Autodesk Fusion 360 part; units mm, degrees
(part 2 of 2)
sketch "Sketch4 (2)" plane through (0, 0, 0) normal (0, 0, 1) x (1, 0, 0)
  circle A0 centre (-53.2335, 49) radius 1.25
  circle A1 centre (-53.2335, -49) radius 1.25
  line L0 (-62.4835, 47.5) -> (-62.4835, -47.5)
  line L1 (-62.4835, -47.5) -> (-57.8585, -47.5)
  line L2 (-57.8585, -47.5) -> (-57.8585, -50.5)
  line L3 (-57.8585, -50.5) -> (-48.6085, -50.5)
  line L4 (-48.6085, -50.5) -> (-48.6085, -47.5)
  line L5 (-48.6085, -47.5) -> (-43.9835, -47.5)
  line L6 (-43.9835, -47.5) -> (-43.9835, -20.41)
  line L7 (-43.9835, -20.41) -> (-46.9835, -20.41)
  line L8 (-46.9835, -20.41) -> (-46.9835, -1.25)
  line L9 (-46.9835, -1.25) -> (-49.8835, -1.25)
  line L10 (-49.8835, -1.25) -> (-49.8835, -2.45)
  line L11 (-49.8835, -2.45) -> (-51.7835, -2.45)
  line L12 (-51.7835, -2.45) -> (-51.7835, -1.25)
  line L13 (-51.7835, -1.25) -> (-53.9835, -1.25)
  line L14 (-53.9835, -1.25) -> (-53.9835, 1.25)
  line L15 (-53.9835, 1.25) -> (-51.7835, 1.25)
  line L16 (-51.7835, 1.25) -> (-51.7835, 2.45)
  line L17 (-51.7835, 2.45) -> (-49.8835, 2.45)
  line L18 (-49.8835, 2.45) -> (-49.8835, 1.25)
  line L19 (-49.8835, 1.25) -> (-46.9835, 1.25)
  line L20 (-46.9835, 1.25) -> (-46.9835, 20.41)
  line L21 (-46.9835, 20.41) -> (-43.9835, 20.41)
  line L22 (-43.9835, 20.41) -> (-43.9835, 47.5)
  line L23 (-43.9835, 47.5) -> (-48.6085, 47.5)
  line L24 (-48.6085, 47.5) -> (-48.6085, 50.5)
  line L25 (-48.6085, 50.5) -> (-57.8585, 50.5)
  line L26 (-57.8585, 50.5) -> (-57.8585, 47.5)
  line L27 (-57.8585, 47.5) -> (-62.4835, 47.5)
  circle A2 centre (-73.7335, 49) radius 1.25
  circle A3 centre (-73.7335, -49) radius 1.25
  line L28 (-82.9835, 47.5) -> (-82.9835, -47.5)
  line L29 (-82.9835, -47.5) -> (-78.3585, -47.5)
  line L30 (-78.3585, -47.5) -> (-78.3585, -50.5)
  line L31 (-78.3585, -50.5) -> (-69.1085, -50.5)
  line L32 (-69.1085, -50.5) -> (-69.1085, -47.5)
  line L33 (-69.1085, -47.5) -> (-64.4835, -47.5)
  line L34 (-64.4835, -47.5) -> (-64.4835, -20.41)
  line L35 (-64.4835, -20.41) -> (-67.4835, -20.41)
  line L36 (-67.4835, -20.41) -> (-67.4835, -1.25)
  line L37 (-67.4835, -1.25) -> (-70.3835, -1.25)
  line L38 (-70.3835, -1.25) -> (-70.3835, -2.45)
  line L39 (-70.3835, -2.45) -> (-72.2835, -2.45)
  line L40 (-72.2835, -2.45) -> (-72.2835, -1.25)
  line L41 (-72.2835, -1.25) -> (-74.4835, -1.25)
  line L42 (-74.4835, -1.25) -> (-74.4835, 1.25)
  line L43 (-74.4835, 1.25) -> (-72.2835, 1.25)
  line L44 (-72.2835, 1.25) -> (-72.2835, 2.45)
  line L45 (-72.2835, 2.45) -> (-70.3835, 2.45)
  line L46 (-70.3835, 2.45) -> (-70.3835, 1.25)
  line L47 (-70.3835, 1.25) -> (-67.4835, 1.25)
  line L48 (-67.4835, 1.25) -> (-67.4835, 20.41)
  line L49 (-67.4835, 20.41) -> (-64.4835, 20.41)
  line L50 (-64.4835, 20.41) -> (-64.4835, 47.5)
  line L51 (-64.4835, 47.5) -> (-69.1085, 47.5)
  line L52 (-69.1085, 47.5) -> (-69.1085, 50.5)
  line L53 (-69.1085, 50.5) -> (-78.3585, 50.5)
  line L54 (-78.3585, 50.5) -> (-78.3585, 47.5)
  line L55 (-78.3585, 47.5) -> (-82.9835, 47.5)
  line L56 (-90.7416, 1.8319) -> (-90.7416, -10.1681)
  line L57 (-90.7416, -10.1681) -> (-97.7416, -10.1681)
  line L58 (-97.7416, -10.1681) -> (-97.7416, 1.8319)
  line L59 (-97.7416, 1.8319) -> (-90.7416, 1.8319)
  line L60 (-85.2416, -36.1681) -> (-85.2416, -13.6681)
  line L61 (-85.2416, -13.6681) -> (-88.2416, -13.6681)
  line L62 (-88.2416, -13.6681) -> (-88.2416, 13.0819)
  line L63 (-88.2416, 13.0819) -> (-91.1416, 13.0819)
  line L64 (-91.1416, 13.0819) -> (-91.1416, 11.8819)
  line L65 (-91.1416, 11.8819) -> (-93.0416, 11.8819)
  line L66 (-93.0416, 11.8819) -> (-93.0416, 13.0819)
  line L67 (-93.0416, 13.0819) -> (-95.2416, 13.0819)
  line L68 (-95.2416, 13.0819) -> (-95.2416, 15.5819)
  line L69 (-95.2416, 15.5819) -> (-93.0416, 15.5819)
  line L70 (-93.0416, 15.5819) -> (-93.0416, 16.7819)
  line L71 (-93.0416, 16.7819) -> (-91.1416, 16.7819)
  line L72 (-91.1416, 16.7819) -> (-91.1416, 15.5819)
  line L73 (-91.1416, 15.5819) -> (-88.2416, 15.5819)
  line L74 (-88.2416, 15.5819) -> (-88.2416, 18.8319)
  line L75 (-88.2416, 18.8319) -> (-85.2416, 18.8319)
  line L76 (-85.2416, 18.8319) -> (-85.2416, 34.3319)
  line L77 (-85.2416, 34.3319) -> (-90.0466, 34.3319)
  line L78 (-90.0466, 34.3319) -> (-90.0466, 31.3547)
  line L79 (-90.0466, 31.3547) -> (-93.2416, 31.3547)
  line L80 (-93.2416, 31.3547) -> (-93.2416, 28.4547)
  line L81 (-93.2416, 28.4547) -> (-92.0416, 28.4547)
  line L82 (-92.0416, 28.4547) -> (-92.0416, 26.5547)
  line L83 (-92.0416, 26.5547) -> (-93.2416, 26.5547)
  line L84 (-93.2416, 26.5547) -> (-93.2416, 24.3547)
  line L85 (-93.2416, 24.3547) -> (-95.7416, 24.3547)
  line L86 (-95.7416, 24.3547) -> (-95.7416, 26.5547)
  line L87 (-95.7416, 26.5547) -> (-96.9416, 26.5547)
  line L88 (-96.9416, 26.5547) -> (-96.9416, 28.4547)
  line L89 (-96.9416, 28.4547) -> (-95.7416, 28.4547)
  line L90 (-95.7416, 28.4547) -> (-95.7416, 31.3547)
  line L91 (-95.7416, 31.3547) -> (-98.9366, 31.3547)
  line L92 (-98.9366, 31.3547) -> (-98.9366, 34.3319)
  line L93 (-98.9366, 34.3319) -> (-103.7416, 34.3319)
  line L94 (-103.7416, 34.3319) -> (-103.7416, -36.1681)
  line L95 (-103.7416, -36.1681) -> (-98.9366, -36.1681)
  line L96 (-98.9366, -36.1681) -> (-98.9366, -33.1681)
  line L97 (-98.9366, -33.1681) -> (-95.7416, -33.1681)
  line L98 (-95.7416, -33.1681) -> (-95.7416, -31.1673)
  line L99 (-95.7416, -31.1673) -> (-96.9416, -31.1673)
  line L100 (-96.9416, -31.1673) -> (-96.9416, -29.2673)
  line L101 (-96.9416, -29.2673) -> (-95.7416, -29.2673)
  line L102 (-95.7416, -29.2673) -> (-95.7416, -27.0673)
  line L103 (-95.7416, -27.0673) -> (-93.2416, -27.0673)
  line L104 (-93.2416, -27.0673) -> (-93.2416, -29.2673)
  line L105 (-93.2416, -29.2673) -> (-92.0416, -29.2673)
  line L106 (-92.0416, -29.2673) -> (-92.0416, -31.1673)
  line L107 (-92.0416, -31.1673) -> (-93.2416, -31.1673)
  line L108 (-93.2416, -31.1673) -> (-93.2416, -33.1681)
  line L109 (-93.2416, -33.1681) -> (-90.0466, -33.1681)
  line L110 (-90.0466, -33.1681) -> (-90.0466, -36.1681)
  line L111 (-90.0466, -36.1681) -> (-85.2416, -36.1681)
  line L112 (-117.2532, 6.84) -> (-108.7532, 6.84)
  line L113 (-108.7532, 6.84) -> (-108.7532, 12.99)
  line L114 (-108.7532, 12.99) -> (-111.6532, 12.99)
  line L115 (-111.6532, 12.99) -> (-111.6532, 11.79)
  line L116 (-111.6532, 11.79) -> (-113.5532, 11.79)
  line L117 (-113.5532, 11.79) -> (-113.5532, 12.99)
  line L118 (-113.5532, 12.99) -> (-115.7532, 12.99)
  line L119 (-115.7532, 12.99) -> (-115.7532, 15.49)
  line L120 (-115.7532, 15.49) -> (-113.5532, 15.49)
  line L121 (-113.5532, 15.49) -> (-113.5532, 16.69)
  line L122 (-113.5532, 16.69) -> (-111.6532, 16.69)
  line L123 (-111.6532, 16.69) -> (-111.6532, 15.49)
  line L124 (-111.6532, 15.49) -> (-108.7532, 15.49)
  line L125 (-108.7532, 15.49) -> (-108.7532, 18.65)
  line L126 (-108.7532, 18.65) -> (-105.7532, 18.65)
  line L127 (-105.7532, 18.65) -> (-105.7532, 34.24)
  line L128 (-105.7532, 34.24) -> (-110.5582, 34.24)
  line L129 (-110.5582, 34.24) -> (-110.5582, 31.3628)
  line L130 (-110.5582, 31.3628) -> (-113.7532, 31.3628)
  line L131 (-113.7532, 31.3628) -> (-113.7532, 28.4628)
  line L132 (-113.7532, 28.4628) -> (-112.5532, 28.4628)
  line L133 (-112.5532, 28.4628) -> (-112.5532, 26.5628)
  line L134 (-112.5532, 26.5628) -> (-113.7532, 26.5628)
  line L135 (-113.7532, 26.5628) -> (-113.7532, 24.3628)
  line L136 (-113.7532, 24.3628) -> (-116.2532, 24.3628)
  line L137 (-116.2532, 24.3628) -> (-116.2532, 26.5628)
  line L138 (-116.2532, 26.5628) -> (-117.4532, 26.5628)
  line L139 (-117.4532, 26.5628) -> (-117.4532, 28.4628)
  line L140 (-117.4532, 28.4628) -> (-116.2532, 28.4628)
  line L141 (-116.2532, 28.4628) -> (-116.2532, 31.3628)
  line L142 (-116.2532, 31.3628) -> (-119.4482, 31.3628)
  line L143 (-119.4482, 31.3628) -> (-119.4482, 34.24)
  line L144 (-119.4482, 34.24) -> (-124.2532, 34.24)
  line L145 (-124.2532, 34.24) -> (-124.2532, -36.26)
  line L146 (-124.2532, -36.26) -> (-119.4482, -36.26)
  line L147 (-119.4482, -36.26) -> (-119.4482, -33.26)
  line L148 (-119.4482, -33.26) -> (-116.2532, -33.26)
  line L149 (-116.2532, -33.26) -> (-116.2532, -31.3593)
  line L150 (-116.2532, -31.3593) -> (-117.4532, -31.3593)
  line L151 (-117.4532, -31.3593) -> (-117.4532, -29.4593)
  line L152 (-117.4532, -29.4593) -> (-116.2532, -29.4593)
  line L153 (-116.2532, -29.4593) -> (-116.2532, -27.2593)
  line L154 (-116.2532, -27.2593) -> (-113.7532, -27.2593)
  line L155 (-113.7532, -27.2593) -> (-113.7532, -29.4593)
  line L156 (-113.7532, -29.4593) -> (-112.5532, -29.4593)
  line L157 (-112.5532, -29.4593) -> (-112.5532, -31.3593)
  line L158 (-112.5532, -31.3593) -> (-113.7532, -31.3593)
  line L159 (-113.7532, -31.3593) -> (-113.7532, -33.26)
  line L160 (-113.7532, -33.26) -> (-110.6037, -33.26)
  line L161 (-110.6037, -33.26) -> (-110.6037, -36.26)
  line L162 (-110.6037, -36.26) -> (-105.7532, -36.26)
  line L163 (-105.7532, -36.26) -> (-105.7532, -13.67)
  line L164 (-105.7532, -13.67) -> (-108.7532, -13.67)
  line L165 (-108.7532, -13.67) -> (-108.7532, -11.86)
  line L166 (-108.7532, -11.86) -> (-117.2532, -11.86)
  line L167 (-117.2532, -11.86) -> (-117.2532, 6.84)
extrude "Extrude7" add sketch "Sketch3 (2)" along normal blind 3 contours A1 L26 L34 L35 | A0 L21 L31 L33 | A1 | A0 | A2 | A2 L27 L38 L39 | A3 | A3 L30 L36 L37 bodies 3 in component "Base"
extrude "Extrude8" cut 4 faces at (-26.4151, 43.1488, -1.5) (27.0849, 43.1488, -1.5) (27.0849, -39.8512, -1.5) (-26.4151, -39.8512, -1.5) along direction (0, 0, -1) blind 3.7 from surface at -1.5 on bodies 3 bodies 3 in component "Base"
component "Internals" placed x (1, 0, 0) y (0, 1, 0) z (0, 0, 1) at (0, 0, 0)
component "Long Side" placed x (1, 0, 0) y (0, 1, 0) z (0, 0, 1) at (0, 0, 0)
component "Base" placed x (1, 0, 0) y (0, 1, 0) z (0, 0, 1) at (0, 0, 0)
component "Short Side" placed x (1, 0, 0) y (0, 1, 0) z (0, 0, 1) at (0, 0, 0)
component "Long Side" placed x (1, 0, 0) y (0, 1, 0) z (0, 0, 1) at (67.5, 0, 0)
component "Short Side v1" placed x (-1, 0, 0) y (0, -1, 0) z (0, 0, 1) at (0, 0, 0)
component "Long Side" placed x (0, 0, 1) y (0, 1, 0) z (-1, 0, 0) at (-45.4835, 0, 42.0165)
component "Long Side" placed x (0, 0, 1) y (0, 1, 0) z (-1, 0, 0) at (-65.9835, 0, 42.0165)
component "Short Side" placed x (0, 1, 0) y (0, 0, -1) z (-1, 0, 0) at (-86.7416, -0.9181, 57.3403)
component "Short Side v1" placed x (0, 1, 0) y (0, 0, -1) z (-1, 0, 0) at (-107.2987, -1.01, 57.7114)
equation "brd_thickness = 1.5 mm"
equation "brd_width = 63.5 mm"
equation "brd_length = 94 mm"
equation "button_side = 12.1 mm"
equation "button_height = 6.4 mm"
equation "slider_width = 3.9 mm"
equation "slider_length = 11.9 mm"
equation "slider_height = 5.2 mm"
equation "screw_dia_lg = 3 mm"
equation "spacer_ff = 4.6 mm"
equation "spacer_ee = 5.2 mm"
equation "spacer_height = 14 mm"
equation "insert_dia = 5.5 mm"
equation "insert_height = 3.7 mm"
equation "brd_tolerance = 1 mm"
equation "d16 = brd_width"
equation "d17 = brd_length"
equation "d18 = brd_thickness"
equation "d22 = screw_dia_lg"
equation "d23 = screw_dia_lg"
equation "d24 = screw_dia_lg"
equation "d25 = screw_dia_lg"
equation "d26 = spacer_height"
equation "d28 = brd_width"
equation "d29 = brd_length"
equation "d30 = brd_thickness"
equation "d34 = button_side"
equation "d35 = button_side"
equation "d36 = button_side"
equation "d37 = button_side"
equation "d38 = button_side"
equation "d39 = button_side"
equation "d40 = button_side"
equation "d41 = button_side"
equation "d42 = slider_width"
equation "d43 = slider_length"
equation "d45 = slider_height"
equation "d47 = button_height"
equation "base_thickness = 6 mm"
equation "acrylic_thickness = 3 mm"
equation "d61 = brd_length + brd_tolerance + ( acrylic_thickness * 2 )"
equation "d62 = brd_thickness + spacer_height"
equation "d63 = 30 mm + ( kerf / 2 )"
equation "d64 = acrylic_thickness"
equation "nut_height = 1.9 mm"
equation "nut_width = 4.9 mm"
equation "screw_base = 13 mm"
equation "screw_sides = 10 mm"
equation "screw_board = 26 mm"
equation "screw_dia_sm = 2.5 mm"
equation "d71 = screw_dia_sm"
equation "d72 = screw_base - base_thickness"
equation "d73 = nut_width"
equation "d74 = nut_height"
equation "d75 = nut_margin"
equation "side_height = brd_thickness + spacer_height + acrylic_thickness"
equation "d77 = acrylic_thickness"
equation "d78 = side_height / 4"
equation "d79 = acrylic_thickness"
equation "d80 = side_height / 4"
equation "d81 = screw_dia_sm"
equation "d82 = acrylic_thickness"
equation "d83 = side_height / 4"
equation "d84 = acrylic_thickness"
equation "d85 = side_height / 4"
equation "d86 = screw_dia_sm"
equation "d87 = acrylic_thickness"
equation "d49_1 = brd_width + brd_tolerance"
equation "d50_1 = brd_length + brd_tolerance"
equation "d53_1 = brd_width + brd_tolerance + ( acrylic_thickness * 2 )"
equation "d54_1 = brd_length + brd_tolerance + ( acrylic_thickness * 2 )"
equation "d55_1 = -brd_thickness"
equation "d56_1 = base_thickness"
equation "d58_1 = -brd_thickness + acrylic_thickness"
equation "d59_1 = base_thickness - acrylic_thickness"
equation "d89 = brd_tolerance / 2"
equation "d90 = screw_dia_sm"
equation "d91 = screw_dia_sm"
equation "d92 = -acrylic_thickness"
equation "d96 = brd_width + ( acrylic_thickness * 2 ) + brd_tolerance"
equation "d97 = brd_thickness + spacer_height + acrylic_thickness"
equation "d98 = acrylic_thickness"
equation "d99 = side_height / 4 + kerf"
equation "d100 = acrylic_thickness"
equation "d101 = side_height / 4 + kerf"
equation "d102 = acrylic_thickness"
equation "d103 = side_height / 4 + kerf"
equation "d104 = acrylic_thickness"
equation "d105 = side_height / 4 + kerf"
equation "d108 = screw_dia_sm"
equation "d113 = screw_sides - acrylic_thickness"
equation "d114 = screw_dia_sm"
equation "d115 = nut_height"
equation "d116 = nut_width"
equation "d117 = nut_margin"
equation "d121 = 12 mm + acrylic_thickness + ( brd_tolerance / 2 )"
equation "d122 = acrylic_thickness"
equation "d123 = 19 mm + acrylic_thickness + ( brd_tolerance / 2 )"
equation "d124 = acrylic_thickness"
equation "d125 = 19 mm + acrylic_thickness + ( brd_tolerance / 2 )"
equation "d126 = acrylic_thickness"
equation "d127 = 12 mm + acrylic_thickness + ( brd_tolerance / 2 )"
equation "d128 = acrylic_thickness"
equation "d129 = screw_dia_sm"
equation "d130 = screw_dia_sm"
equation "post_offset_x = 6 mm"
equation "post_offset_y = 5.5 mm"
equation "d133 = insert_dia * 2"
equation "d134 = post_offset_x"
equation "d135 = post_offset_y"
equation "d136 = insert_dia"
equation "port_margin1 = 29 mm + acrylic_thickness + ( brd_tolerance / 2 )"
equation "port_margin2 = 22.5 mm + acrylic_thickness + ( brd_tolerance / 2 )"
equation "port_x = total_width - port_margin1 - port_margin2"
equation "backup_port_margin = 22.4 mm"
equation "backup_port_x = brd_width - ( backup_port_margin * 2 )"
equation "backup_port_y = 8.5 mm"
equation "port_marginy = 4.5 mm - brd_thickness"
equation "port_y = 7 mm"
equation "d152 = 15.5 mm + 4.5 mm"
equation "d153 = 12 mm + acrylic_thickness + ( brd_tolerance / 2 ) + ( kerf / 2 )"
equation "d154 = 19 mm + acrylic_thickness + ( brd_tolerance / 2 ) + ( kerf / 2 )"
equation "d155 = screw_base - base_thickness"
equation "d156 = nut_width"
equation "d157 = nut_height"
equation "d159 = port_x"
equation "d160 = port_y"
equation "total_width = brd_width + ( acrylic_thickness * 2 ) + brd_tolerance"
equation "d162 = port_margin2"
equation "d96_1 = brd_width_1 + ( acrylic_thickness_1 * 2 ) + brd_tolerance_1"
equation "d97_1 = brd_thickness_1 + spacer_height_1 + acrylic_thickness_1"
equation "d98_1 = acrylic_thickness_1"
equation "d99_1 = side_height_1 / 4 + kerf"
equation "d100_1 = acrylic_thickness_1"
equation "d101_1 = side_height_1 / 4 + kerf"
equation "d102_1 = acrylic_thickness_1"
equation "d103_1 = side_height_1 / 4 + kerf"
equation "d104_1 = acrylic_thickness_1"
equation "d105_1 = side_height_1 / 4 + kerf"
equation "d108_1 = screw_dia_sm_1"
equation "d113_1 = screw_sides_1 - acrylic_thickness_1"
equation "d114_1 = screw_dia_sm_1"
equation "d115_1 = nut_height_1"
equation "d116_1 = nut_width_1"
equation "d117_1 = nut_margin"
equation "d152_1 = 15.5 mm + 4.5 mm"
equation "d153_1 = 12 mm + acrylic_thickness_1 + ( brd_tolerance_1 / 2 ) + ( kerf / 2 )"
equation "d154_1 = 19 mm + acrylic_thickness_1 + ( brd_tolerance_1 / 2 ) + ( kerf / 2 )"
equation "d155_1 = screw_base_1 - base_thickness_1"
equation "d156_1 = nut_width_1"
equation "d157_1 = nut_height_1"
equation "brd_thickness_1 = brd_thickness"
equation "brd_width_1 = brd_width"
equation "spacer_height_1 = spacer_height"
equation "brd_tolerance_1 = brd_tolerance"
equation "base_thickness_1 = base_thickness"
equation "acrylic_thickness_1 = acrylic_thickness"
equation "nut_height_1 = nut_height"
equation "nut_width_1 = nut_width"
equation "screw_base_1 = screw_base"
equation "screw_sides_1 = screw_sides"
equation "screw_dia_sm_1 = screw_dia_sm"
equation "side_height_1 = side_height"
equation "d172 = backup_port_x"
equation "d173 = backup_port_y"
equation "d174 = backup_port_margin + 2 mm"
equation "nut_margin = acrylic_thickness - 0.1 mm"
equation "kerf = 0.18 mm"
equation "d181 = brd_tolerance / 2"
equation "d182 = acrylic_thickness"
equation "d184 = nut_margin"
equation "d185 = screw_dia_sm"
equation "d186 = screw_dia_sm"
equation "d188 = acrylic_thickness"
equation "d189 = nut_margin"
equation "d190 = brd_tolerance / 2"
equation "d191 = acrylic_thickness"
equation "d193 = acrylic_thickness"
equation "d195 = acrylic_thickness - brd_thickness"
equation "d196 = -insert_height"
